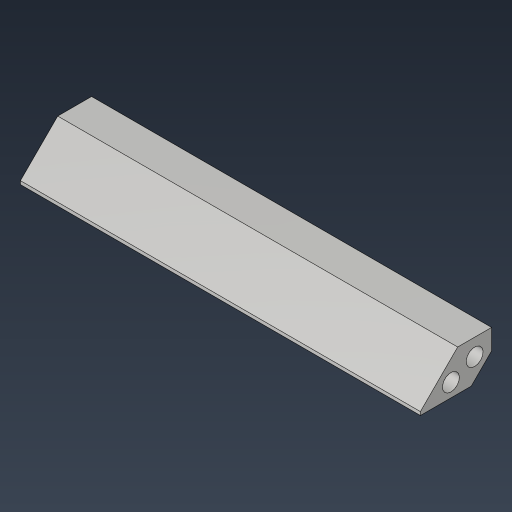
# Autodesk Inventor part: Chip Schaufel Mitte
Saved by Autodesk Inventor 2023.1 (Build 271208000, 208)
## iProperties
Part Number: Chip Schaufel Mitte
Material: Aluminium 6061
Document SubType Name: Modeling
Designer: rYan
Mass: 6.57298 g
Surface Area: 19.3489 cm^2
Volume: 2.43444 cm^3
Density: 2.7 g/cm^3
Appearance: Aluminium - flach
Author: rYan
Autodesk Inventor part; units mm, degrees
ref_plane "YZ Plane" through (0, 0, 0) normal (1, 0, 0) x (0, 1, 0)
ref_plane "XZ Plane" through (0, 0, 0) normal (0, 1, 0) x (-1, 0, 0)
ref_plane "XY Plane" through (0, 0, 0) normal (0, 0, 1) x (1, 0, 0)
sketch "Skizze1" plane through (0, 0, 0) normal (1, 0, 0) x (0, 1, 0)
  line L0 (-5, 6) -> (-10.5, 0.5)
  line L1 (-10.5, 0) -> (0, 0)
  line L2 (0, 0) -> (0, 6)
  line L3 (0, 6) -> (-5, 6)
  line L4 (-10.5, 0) -> (-10.5, 0.5)
  dimension "d35" = 45
  dimension "d54" = 6
  dimension "d55" = 0.5
  dimension "d56" = 10.5
  constraints: 10 end point, 2 perpendicular, 1 coincident, 1 horizontal, 1 vertical
  measures "d35" angle of L1 L0
  measures "d54" distance from line of L1 L0.start
  measures "d55" distance of L1.start L0.end
  measures "d56" distance from line of L1.start L2
extrude "Extrusion1" add sketch "Skizze1" along normal mid plane 59
fillet "Rundung2" [suppressed]
sketch "Skizze5" plane through (29.5, 0, 0) normal (1, 0, 0) x (0, 0, -1)
  line L0 (-7.2, 0) -> (1.2, 0) projected
  line L1 (0, -12.6) -> (0, 2.1) projected
  point P0 (0, 0)
  point P1 (-3.7, -4)
  dimension "d36" = 3.7
  dimension "d37" = 4
  measures "d36" distance from line of point (-3.7, -4) L1
  measures "d37" distance from line of L0 point (-3.7, -4)
hole "Bohrung3" [suppressed]
sketch "Skizze6" plane through (29.5, 0, 0) normal (1, 0, 0) x (0, 0, -1)
  line L0 (-7.2, 0) -> (1.2, 0) projected
  line L1 (0, -12.6) -> (0, 2.1) projected
  point P0 (0, 0)
  point P1 (-3.5, -2.5)
  point P2 (-2, -6)
  dimension "d45" = 3.5
  dimension "d46" = 2.5
  dimension "d65" = 1.5
  dimension "d66" = 3.5
  measures "d45" distance from line of point (-3.5, -2.5) L1
  measures "d46" distance from line of L0 point (-3.5, -2.5)
  measures "d65" horizontal distance of point (-2, -6) point (-3.5, -2.5)
  measures "d66" vertical distance of point (-2, -6) point (-3.5, -2.5)
hole "Bohrung4" at (29.5, -2.5, 3.5) at (29.5, -6, 2) direction (-1, 0, 0) diameter 2.5 depth 6.1 tip angle 118
mirror "Spiegeln1" about plane through (0, 0, 0) normal (1, 0, 0) of "Bohrung4"
sketch "Skizze7" plane through (-29.5, -5, 6) normal (0, 0, 1) x (1, 0, 0)
  line L0 (0, 0) -> (59, 0) projected
  line L1 (59, 5) -> (59, 0) projected
  line L2 (59, 5) -> (0, 5) projected
  line L3 (0, 0) -> (0, 5) projected
  line L4 (0, 0) -> (0, 5) construction
  line L5 (0, 2.5) -> (59, 2.5) construction
  line L6 (29.5, 5) -> (29.5, 0) construction
  line L7 (0, 0) -> (59, 0) construction
  point P0 (15.5, 2.5)
  point P1 (43.5, 2.5)
  point P2 (29.5, 2.5)
  dimension "d57" = 14
  constraints: 4 end point, 4 midpoint, 2 point on line, 1 symmetric about line
  measures "d57" distance from line of L6 point (15.5, 2.5)
hole "Bohrung5" [suppressed]
chamfer "Fase2" distance 3 angle 45 1 edges at (0, 0, 0)
